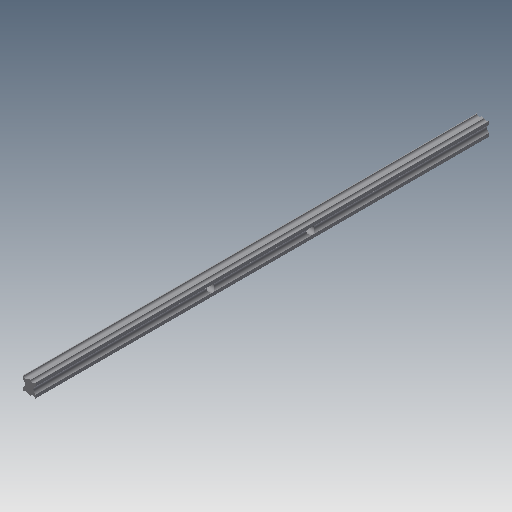
# Autodesk Inventor part: SAR340-40_r
Saved by Autodesk Inventor 2020 (Build 240168000, 168)
## iProperties
Created: 2019-11-23
Part Number: SAR340-40_r
Material: Generic
Catalog Web Link: www.cadenas.de
Description: SAR3_rail-Slide Rails - Aluminum Alloy - Three - Step Slide Rails
Vendor: MISUMI
Document SubType Name: Modeling
Designer: psadmin
Manufacturer: MISUMI
Mass: 40.319 g
Surface Area: 227.079 cm^2
Volume: 40.319 cm^3
Density: 1 g/cm^3
Appearance: PSOLRGB-192-192-192
Category: PARTsolutions
Company: MISUMI
PSOL_IDENT_0: {$CADENAS_DATA\23d-libs\misumi\metric\07_slide_rails\sar3_series\sar3_rail.prj},167 {VTYP=3D},{NB=SA
PSOL_IDENT_1: R340-40_r},{LINA=SAR340-40},{NN=SAR3_rail},{DATE=17.04.2019 06:32:22},{GEOMDATE=16.04.2019 09:30:43}
PSOL_IDENT_2: ,{VERSION=},{LINEID=10},{WBVAR=NO},{WBNUMERIC=NO}  {NB=SAR340-40_r},{LINA=SAR340-40},{KT=DUMMY},{PN=
PSOL_IDENT_3: SAR340-40},{TYPE=SAR340},{MAT1=Aluminum Alloy},{ST1=Clear Anodizing},{MAT2=Aluminum Alloy},{ST2=Clea
PSOL_IDENT_4: r Anodizing},{MAT3=Steel},{NO=40},{RL=400},{TD=460},{A=185},{B=370},{C=185},{D=370},{RLO=147},{BA=36
PSOL_IDENT_5: },{E=156.000},{F=88.000}
NN: SAR3_rail
NT: Slide Rails - Aluminum Alloy - Three - Step Slide Rails
NB: SAR340-40_r
NBSYN: $PN._r
LINA: SAR340-40
PN: SAR340-40
MAT1: Aluminum Alloy
ST1: Clear Anodizing
MAT2: Aluminum Alloy
ST2: Clear Anodizing
MAT3: Steel
NO: 40
RLO: 147
SUPPLIER: MISUMI
ARTICLENO: SAR340-40_r
BOMINFO: SAR340-40
CREATOR: CADENAS GmbH
Title: SAR340-40
Author: Cadenas PARTsolutions
Comments: Slide Rails - Aluminum Alloy - Three - Step Slide Rails
Autodesk Inventor part; units mm, degrees
sketch "_____1" plane through (0, 0, 0) normal (0, 0, 1) x (1, 0, 0)
  arc A0 (0, 0.2) -> (0.2, 0) centre (0.2, 0.2) ccw
  line L0 (0.2, 0) -> (0.5141, 0)
  arc A1 (0.5141, 0) -> (0.708, 0.151) centre (0.5141, 0.2) ccw
  arc A2 (4.392, 0.151) -> (0.708, 0.151) centre (2.55, -0.315) ccw
  arc A3 (4.392, 0.151) -> (4.5859, 0) centre (4.5859, 0.2) ccw
  line L1 (4.5859, 0) -> (6.8141, 0)
  arc A4 (6.8141, 0) -> (7.008, 0.151) centre (6.8141, 0.2) ccw
  arc A5 (10.692, 0.151) -> (7.008, 0.151) centre (8.85, -0.315) ccw
  arc A6 (10.692, 0.151) -> (10.8859, 0) centre (10.8859, 0.2) ccw
  line L2 (10.8859, 0) -> (11.2, 0)
  arc A7 (11.2, 0) -> (11.4, 0.2) centre (11.2, 0.2) ccw
  line L3 (11.4, 0.2) -> (11.4, 2.838)
  arc A8 (11.4, 2.838) -> (11.2882, 3.0174) centre (11.2, 2.838) ccw
  arc A9 (11.2882, 9.0826) -> (11.2882, 3.0174) centre (12.7793, 6.05) ccw
  arc A10 (11.2882, 9.0826) -> (11.4, 9.262) centre (11.2, 9.262) ccw
  line L4 (11.4, 9.262) -> (11.4, 11.9)
  arc A11 (11.4, 11.9) -> (11.2, 12.1) centre (11.2, 11.9) ccw
  line L5 (11.2, 12.1) -> (10.8859, 12.1)
  arc A12 (10.8859, 12.1) -> (10.692, 11.949) centre (10.8859, 11.9) ccw
  arc A13 (7.008, 11.949) -> (10.692, 11.949) centre (8.85, 12.415) ccw
  arc A14 (7.008, 11.949) -> (6.8141, 12.1) centre (6.8141, 11.9) ccw
  line L6 (6.8141, 12.1) -> (4.5859, 12.1)
  arc A15 (4.5859, 12.1) -> (4.392, 11.949) centre (4.5859, 11.9) ccw
  arc A16 (0.708, 11.949) -> (4.392, 11.949) centre (2.55, 12.415) ccw
  arc A17 (0.708, 11.949) -> (0.5141, 12.1) centre (0.5141, 11.9) ccw
  line L7 (0.5141, 12.1) -> (0.2, 12.1)
  arc A18 (0.2, 12.1) -> (0, 11.9) centre (0.2, 11.9) ccw
  line L8 (0, 11.9) -> (0, 9.262)
  arc A19 (0, 9.262) -> (0.1118, 9.0826) centre (0.2, 9.262) ccw
  arc A20 (0.1118, 3.0174) -> (0.1118, 9.0826) centre (-1.3793, 6.05) ccw
  arc A21 (0.1118, 3.0174) -> (0, 2.838) centre (0.2, 2.838) ccw
  line L9 (0, 2.838) -> (0, 0.2)
  constraints: 44 point on circle, 22 centre point, 20 end point
extrude "Extrusion1" add sketch "_____1" along normal blind 400
sketch "Sketch_3" plane through (0, 0, 156) normal (0, 0, 1) x (1, 0, 0)
  line L0 (11.4, 6.05) -> (0, 6.05)
  line L1 (0, 6.05) -> (0, 9.3)
  line L2 (0, 9.3) -> (11.4, 9.3)
  line L3 (11.4, 9.3) -> (11.4, 6.05)
  line L4 (11.4, 6.05) -> (0, 6.05)
  constraints: 10 end point
revolve "Revolution1" cut sketch "Sketch_3" angle 360 about axis through (11.4, 6.05, 156) along (1, 0, 0)
pattern_linear "Rectangular Pattern1" count 2 spacing 88 along (0, 0, 1) of "Revolution1"
ref_plane "to_ball1_1_XY" through (2.55, -0.4, 268.4) normal (0, 1, 0) x (1, 0, 0)
ref_plane "to_ball1_1_YZ" through (2.55, -0.4, 268.4) normal (1, 0, 0) x (0, 0, -1)
ref_plane "to_ball1_1_ZX" through (2.55, -0.4, 268.4) normal (0, 0, -1) x (0, 1, 0)
ref_plane "to_ball1_10_XY" through (2.55, -0.4, 234.2) normal (0, 1, 0) x (1, 0, 0)
ref_plane "to_ball1_10_YZ" through (2.55, -0.4, 234.2) normal (1, 0, 0) x (0, 0, -1)
ref_plane "to_ball1_10_ZX" through (2.55, -0.4, 234.2) normal (0, 0, -1) x (0, 1, 0)
ref_plane "to_ball1_11_XY" through (2.55, -0.4, 230.4) normal (0, 1, 0) x (1, 0, 0)
ref_plane "to_ball1_11_YZ" through (2.55, -0.4, 230.4) normal (1, 0, 0) x (0, 0, -1)
ref_plane "to_ball1_11_ZX" through (2.55, -0.4, 230.4) normal (0, 0, -1) x (0, 1, 0)
ref_plane "to_ball1_12_XY" through (2.55, -0.4, 226.6) normal (0, 1, 0) x (1, 0, 0)
ref_plane "to_ball1_12_YZ" through (2.55, -0.4, 226.6) normal (1, 0, 0) x (0, 0, -1)
ref_plane "to_ball1_12_ZX" through (2.55, -0.4, 226.6) normal (0, 0, -1) x (0, 1, 0)
ref_plane "to_ball1_13_XY" through (2.55, -0.4, 222.8) normal (0, 1, 0) x (1, 0, 0)
ref_plane "to_ball1_13_YZ" through (2.55, -0.4, 222.8) normal (1, 0, 0) x (0, 0, -1)
ref_plane "to_ball1_13_ZX" through (2.55, -0.4, 222.8) normal (0, 0, -1) x (0, 1, 0)
ref_plane "to_ball1_14_XY" through (2.55, -0.4, 219) normal (0, 1, 0) x (1, 0, 0)
ref_plane "to_ball1_14_YZ" through (2.55, -0.4, 219) normal (1, 0, 0) x (0, 0, -1)
ref_plane "to_ball1_14_ZX" through (2.55, -0.4, 219) normal (0, 0, -1) x (0, 1, 0)
ref_plane "to_ball1_15_XY" through (2.55, -0.4, 215.2) normal (0, 1, 0) x (1, 0, 0)
ref_plane "to_ball1_15_YZ" through (2.55, -0.4, 215.2) normal (1, 0, 0) x (0, 0, -1)
ref_plane "to_ball1_15_ZX" through (2.55, -0.4, 215.2) normal (0, 0, -1) x (0, 1, 0)
ref_plane "to_ball1_16_XY" through (2.55, -0.4, 211.4) normal (0, 1, 0) x (1, 0, 0)
ref_plane "to_ball1_16_YZ" through (2.55, -0.4, 211.4) normal (1, 0, 0) x (0, 0, -1)
ref_plane "to_ball1_16_ZX" through (2.55, -0.4, 211.4) normal (0, 0, -1) x (0, 1, 0)
ref_plane "to_ball1_17_XY" through (2.55, -0.4, 207.6) normal (0, 1, 0) x (1, 0, 0)
ref_plane "to_ball1_17_YZ" through (2.55, -0.4, 207.6) normal (1, 0, 0) x (0, 0, -1)
ref_plane "to_ball1_17_ZX" through (2.55, -0.4, 207.6) normal (0, 0, -1) x (0, 1, 0)
ref_plane "to_ball1_18_XY" through (2.55, -0.4, 203.8) normal (0, 1, 0) x (1, 0, 0)
ref_plane "to_ball1_18_YZ" through (2.55, -0.4, 203.8) normal (1, 0, 0) x (0, 0, -1)
ref_plane "to_ball1_18_ZX" through (2.55, -0.4, 203.8) normal (0, 0, -1) x (0, 1, 0)
ref_plane "to_ball1_19_XY" through (2.55, -0.4, 200) normal (0, 1, 0) x (1, 0, 0)
ref_plane "to_ball1_19_YZ" through (2.55, -0.4, 200) normal (1, 0, 0) x (0, 0, -1)
ref_plane "to_ball1_19_ZX" through (2.55, -0.4, 200) normal (0, 0, -1) x (0, 1, 0)
ref_plane "to_ball1_2_XY" through (2.55, -0.4, 264.6) normal (0, 1, 0) x (1, 0, 0)
ref_plane "to_ball1_2_YZ" through (2.55, -0.4, 264.6) normal (1, 0, 0) x (0, 0, -1)
ref_plane "to_ball1_2_ZX" through (2.55, -0.4, 264.6) normal (0, 0, -1) x (0, 1, 0)
ref_plane "to_ball1_20_XY" through (2.55, -0.4, 196.2) normal (0, 1, 0) x (1, 0, 0)
ref_plane "to_ball1_20_YZ" through (2.55, -0.4, 196.2) normal (1, 0, 0) x (0, 0, -1)
ref_plane "to_ball1_20_ZX" through (2.55, -0.4, 196.2) normal (0, 0, -1) x (0, 1, 0)
ref_plane "to_ball1_21_XY" through (2.55, -0.4, 192.4) normal (0, 1, 0) x (1, 0, 0)
ref_plane "to_ball1_21_YZ" through (2.55, -0.4, 192.4) normal (1, 0, 0) x (0, 0, -1)
ref_plane "to_ball1_21_ZX" through (2.55, -0.4, 192.4) normal (0, 0, -1) x (0, 1, 0)
ref_plane "to_ball1_22_XY" through (2.55, -0.4, 188.6) normal (0, 1, 0) x (1, 0, 0)
ref_plane "to_ball1_22_YZ" through (2.55, -0.4, 188.6) normal (1, 0, 0) x (0, 0, -1)
ref_plane "to_ball1_22_ZX" through (2.55, -0.4, 188.6) normal (0, 0, -1) x (0, 1, 0)
ref_plane "to_ball1_23_XY" through (2.55, -0.4, 184.8) normal (0, 1, 0) x (1, 0, 0)
ref_plane "to_ball1_23_YZ" through (2.55, -0.4, 184.8) normal (1, 0, 0) x (0, 0, -1)
ref_plane "to_ball1_23_ZX" through (2.55, -0.4, 184.8) normal (0, 0, -1) x (0, 1, 0)
ref_plane "to_ball1_24_XY" through (2.55, -0.4, 181) normal (0, 1, 0) x (1, 0, 0)
ref_plane "to_ball1_24_YZ" through (2.55, -0.4, 181) normal (1, 0, 0) x (0, 0, -1)
ref_plane "to_ball1_24_ZX" through (2.55, -0.4, 181) normal (0, 0, -1) x (0, 1, 0)
ref_plane "to_ball1_25_XY" through (2.55, -0.4, 177.2) normal (0, 1, 0) x (1, 0, 0)
ref_plane "to_ball1_25_YZ" through (2.55, -0.4, 177.2) normal (1, 0, 0) x (0, 0, -1)
ref_plane "to_ball1_25_ZX" through (2.55, -0.4, 177.2) normal (0, 0, -1) x (0, 1, 0)
ref_plane "to_ball1_26_XY" through (2.55, -0.4, 173.4) normal (0, 1, 0) x (1, 0, 0)
ref_plane "to_ball1_26_YZ" through (2.55, -0.4, 173.4) normal (1, 0, 0) x (0, 0, -1)
ref_plane "to_ball1_26_ZX" through (2.55, -0.4, 173.4) normal (0, 0, -1) x (0, 1, 0)
ref_plane "to_ball1_27_XY" through (2.55, -0.4, 169.6) normal (0, 1, 0) x (1, 0, 0)
ref_plane "to_ball1_27_YZ" through (2.55, -0.4, 169.6) normal (1, 0, 0) x (0, 0, -1)
ref_plane "to_ball1_27_ZX" through (2.55, -0.4, 169.6) normal (0, 0, -1) x (0, 1, 0)
ref_plane "to_ball1_28_XY" through (2.55, -0.4, 165.8) normal (0, 1, 0) x (1, 0, 0)
ref_plane "to_ball1_28_YZ" through (2.55, -0.4, 165.8) normal (1, 0, 0) x (0, 0, -1)
ref_plane "to_ball1_28_ZX" through (2.55, -0.4, 165.8) normal (0, 0, -1) x (0, 1, 0)
ref_plane "to_ball1_29_XY" through (2.55, -0.4, 162) normal (0, 1, 0) x (1, 0, 0)
ref_plane "to_ball1_29_YZ" through (2.55, -0.4, 162) normal (1, 0, 0) x (0, 0, -1)
ref_plane "to_ball1_29_ZX" through (2.55, -0.4, 162) normal (0, 0, -1) x (0, 1, 0)
ref_plane "to_ball1_3_XY" through (2.55, -0.4, 260.8) normal (0, 1, 0) x (1, 0, 0)
ref_plane "to_ball1_3_YZ" through (2.55, -0.4, 260.8) normal (1, 0, 0) x (0, 0, -1)
ref_plane "to_ball1_3_ZX" through (2.55, -0.4, 260.8) normal (0, 0, -1) x (0, 1, 0)
ref_plane "to_ball1_30_XY" through (2.55, -0.4, 158.2) normal (0, 1, 0) x (1, 0, 0)
ref_plane "to_ball1_30_YZ" through (2.55, -0.4, 158.2) normal (1, 0, 0) x (0, 0, -1)
ref_plane "to_ball1_30_ZX" through (2.55, -0.4, 158.2) normal (0, 0, -1) x (0, 1, 0)
ref_plane "to_ball1_31_XY" through (2.55, -0.4, 154.4) normal (0, 1, 0) x (1, 0, 0)
ref_plane "to_ball1_31_YZ" through (2.55, -0.4, 154.4) normal (1, 0, 0) x (0, 0, -1)
ref_plane "to_ball1_31_ZX" through (2.55, -0.4, 154.4) normal (0, 0, -1) x (0, 1, 0)
ref_plane "to_ball1_32_XY" through (2.55, -0.4, 150.6) normal (0, 1, 0) x (1, 0, 0)
ref_plane "to_ball1_32_YZ" through (2.55, -0.4, 150.6) normal (1, 0, 0) x (0, 0, -1)
ref_plane "to_ball1_32_ZX" through (2.55, -0.4, 150.6) normal (0, 0, -1) x (0, 1, 0)
ref_plane "to_ball1_33_XY" through (2.55, -0.4, 146.8) normal (0, 1, 0) x (1, 0, 0)
ref_plane "to_ball1_33_YZ" through (2.55, -0.4, 146.8) normal (1, 0, 0) x (0, 0, -1)
ref_plane "to_ball1_33_ZX" through (2.55, -0.4, 146.8) normal (0, 0, -1) x (0, 1, 0)
ref_plane "to_ball1_34_XY" through (2.55, -0.4, 143) normal (0, 1, 0) x (1, 0, 0)
ref_plane "to_ball1_34_YZ" through (2.55, -0.4, 143) normal (1, 0, 0) x (0, 0, -1)
ref_plane "to_ball1_34_ZX" through (2.55, -0.4, 143) normal (0, 0, -1) x (0, 1, 0)
ref_plane "to_ball1_35_XY" through (2.55, -0.4, 139.2) normal (0, 1, 0) x (1, 0, 0)
ref_plane "to_ball1_35_YZ" through (2.55, -0.4, 139.2) normal (1, 0, 0) x (0, 0, -1)
ref_plane "to_ball1_35_ZX" through (2.55, -0.4, 139.2) normal (0, 0, -1) x (0, 1, 0)
ref_plane "to_ball1_36_XY" through (2.55, -0.4, 135.4) normal (0, 1, 0) x (1, 0, 0)
ref_plane "to_ball1_36_YZ" through (2.55, -0.4, 135.4) normal (1, 0, 0) x (0, 0, -1)
ref_plane "to_ball1_36_ZX" through (2.55, -0.4, 135.4) normal (0, 0, -1) x (0, 1, 0)
ref_plane "to_ball1_37_XY" through (2.55, -0.4, 131.6) normal (0, 1, 0) x (1, 0, 0)
ref_plane "to_ball1_37_YZ" through (2.55, -0.4, 131.6) normal (1, 0, 0) x (0, 0, -1)
ref_plane "to_ball1_37_ZX" through (2.55, -0.4, 131.6) normal (0, 0, -1) x (0, 1, 0)
ref_plane "to_ball1_4_XY" through (2.55, -0.4, 257) normal (0, 1, 0) x (1, 0, 0)
ref_plane "to_ball1_4_YZ" through (2.55, -0.4, 257) normal (1, 0, 0) x (0, 0, -1)
ref_plane "to_ball1_4_ZX" through (2.55, -0.4, 257) normal (0, 0, -1) x (0, 1, 0)
ref_plane "to_ball1_5_XY" through (2.55, -0.4, 253.2) normal (0, 1, 0) x (1, 0, 0)
ref_plane "to_ball1_5_YZ" through (2.55, -0.4, 253.2) normal (1, 0, 0) x (0, 0, -1)
ref_plane "to_ball1_5_ZX" through (2.55, -0.4, 253.2) normal (0, 0, -1) x (0, 1, 0)
ref_plane "to_ball1_6_XY" through (2.55, -0.4, 249.4) normal (0, 1, 0) x (1, 0, 0)
ref_plane "to_ball1_6_YZ" through (2.55, -0.4, 249.4) normal (1, 0, 0) x (0, 0, -1)
ref_plane "to_ball1_6_ZX" through (2.55, -0.4, 249.4) normal (0, 0, -1) x (0, 1, 0)
ref_plane "to_ball1_7_XY" through (2.55, -0.4, 245.6) normal (0, 1, 0) x (1, 0, 0)
ref_plane "to_ball1_7_YZ" through (2.55, -0.4, 245.6) normal (1, 0, 0) x (0, 0, -1)
ref_plane "to_ball1_7_ZX" through (2.55, -0.4, 245.6) normal (0, 0, -1) x (0, 1, 0)
ref_plane "to_ball1_8_XY" through (2.55, -0.4, 241.8) normal (0, 1, 0) x (1, 0, 0)
ref_plane "to_ball1_8_YZ" through (2.55, -0.4, 241.8) normal (1, 0, 0) x (0, 0, -1)
ref_plane "to_ball1_8_ZX" through (2.55, -0.4, 241.8) normal (0, 0, -1) x (0, 1, 0)
ref_plane "to_ball1_9_XY" through (2.55, -0.4, 238) normal (0, 1, 0) x (1, 0, 0)
ref_plane "to_ball1_9_YZ" through (2.55, -0.4, 238) normal (1, 0, 0) x (0, 0, -1)
ref_plane "to_ball1_9_ZX" through (2.55, -0.4, 238) normal (0, 0, -1) x (0, 1, 0)
ref_plane "to_ball2_1_XY" through (8.85, -0.4, 268.4) normal (0, 1, 0) x (1, 0, 0)
ref_plane "to_ball2_1_YZ" through (8.85, -0.4, 268.4) normal (1, 0, 0) x (0, 0, -1)
ref_plane "to_ball2_1_ZX" through (8.85, -0.4, 268.4) normal (0, 0, -1) x (0, 1, 0)
ref_plane "to_ball2_10_XY" through (8.85, -0.4, 234.2) normal (0, 1, 0) x (1, 0, 0)
ref_plane "to_ball2_10_YZ" through (8.85, -0.4, 234.2) normal (1, 0, 0) x (0, 0, -1)
ref_plane "to_ball2_10_ZX" through (8.85, -0.4, 234.2) normal (0, 0, -1) x (0, 1, 0)
ref_plane "to_ball2_11_XY" through (8.85, -0.4, 230.4) normal (0, 1, 0) x (1, 0, 0)
ref_plane "to_ball2_11_YZ" through (8.85, -0.4, 230.4) normal (1, 0, 0) x (0, 0, -1)
ref_plane "to_ball2_11_ZX" through (8.85, -0.4, 230.4) normal (0, 0, -1) x (0, 1, 0)
ref_plane "to_ball2_12_XY" through (8.85, -0.4, 226.6) normal (0, 1, 0) x (1, 0, 0)
ref_plane "to_ball2_12_YZ" through (8.85, -0.4, 226.6) normal (1, 0, 0) x (0, 0, -1)
ref_plane "to_ball2_12_ZX" through (8.85, -0.4, 226.6) normal (0, 0, -1) x (0, 1, 0)
ref_plane "to_ball2_13_XY" through (8.85, -0.4, 222.8) normal (0, 1, 0) x (1, 0, 0)
ref_plane "to_ball2_13_YZ" through (8.85, -0.4, 222.8) normal (1, 0, 0) x (0, 0, -1)
ref_plane "to_ball2_13_ZX" through (8.85, -0.4, 222.8) normal (0, 0, -1) x (0, 1, 0)
ref_plane "to_ball2_14_XY" through (8.85, -0.4, 219) normal (0, 1, 0) x (1, 0, 0)
ref_plane "to_ball2_14_YZ" through (8.85, -0.4, 219) normal (1, 0, 0) x (0, 0, -1)
ref_plane "to_ball2_14_ZX" through (8.85, -0.4, 219) normal (0, 0, -1) x (0, 1, 0)
ref_plane "to_ball2_15_XY" through (8.85, -0.4, 215.2) normal (0, 1, 0) x (1, 0, 0)
ref_plane "to_ball2_15_YZ" through (8.85, -0.4, 215.2) normal (1, 0, 0) x (0, 0, -1)
ref_plane "to_ball2_15_ZX" through (8.85, -0.4, 215.2) normal (0, 0, -1) x (0, 1, 0)
ref_plane "to_ball2_16_XY" through (8.85, -0.4, 211.4) normal (0, 1, 0) x (1, 0, 0)
ref_plane "to_ball2_16_YZ" through (8.85, -0.4, 211.4) normal (1, 0, 0) x (0, 0, -1)
ref_plane "to_ball2_16_ZX" through (8.85, -0.4, 211.4) normal (0, 0, -1) x (0, 1, 0)
ref_plane "to_ball2_17_XY" through (8.85, -0.4, 207.6) normal (0, 1, 0) x (1, 0, 0)
ref_plane "to_ball2_17_YZ" through (8.85, -0.4, 207.6) normal (1, 0, 0) x (0, 0, -1)
ref_plane "to_ball2_17_ZX" through (8.85, -0.4, 207.6) normal (0, 0, -1) x (0, 1, 0)
ref_plane "to_ball2_18_XY" through (8.85, -0.4, 203.8) normal (0, 1, 0) x (1, 0, 0)
ref_plane "to_ball2_18_YZ" through (8.85, -0.4, 203.8) normal (1, 0, 0) x (0, 0, -1)
ref_plane "to_ball2_18_ZX" through (8.85, -0.4, 203.8) normal (0, 0, -1) x (0, 1, 0)
ref_plane "to_ball2_19_XY" through (8.85, -0.4, 200) normal (0, 1, 0) x (1, 0, 0)
ref_plane "to_ball2_19_YZ" through (8.85, -0.4, 200) normal (1, 0, 0) x (0, 0, -1)
ref_plane "to_ball2_19_ZX" through (8.85, -0.4, 200) normal (0, 0, -1) x (0, 1, 0)
ref_plane "to_ball2_2_XY" through (8.85, -0.4, 264.6) normal (0, 1, 0) x (1, 0, 0)
ref_plane "to_ball2_2_YZ" through (8.85, -0.4, 264.6) normal (1, 0, 0) x (0, 0, -1)
ref_plane "to_ball2_2_ZX" through (8.85, -0.4, 264.6) normal (0, 0, -1) x (0, 1, 0)
ref_plane "to_ball2_20_XY" through (8.85, -0.4, 196.2) normal (0, 1, 0) x (1, 0, 0)
ref_plane "to_ball2_20_YZ" through (8.85, -0.4, 196.2) normal (1, 0, 0) x (0, 0, -1)
ref_plane "to_ball2_20_ZX" through (8.85, -0.4, 196.2) normal (0, 0, -1) x (0, 1, 0)
ref_plane "to_ball2_21_XY" through (8.85, -0.4, 192.4) normal (0, 1, 0) x (1, 0, 0)
ref_plane "to_ball2_21_YZ" through (8.85, -0.4, 192.4) normal (1, 0, 0) x (0, 0, -1)
ref_plane "to_ball2_21_ZX" through (8.85, -0.4, 192.4) normal (0, 0, -1) x (0, 1, 0)
ref_plane "to_ball2_22_XY" through (8.85, -0.4, 188.6) normal (0, 1, 0) x (1, 0, 0)
ref_plane "to_ball2_22_YZ" through (8.85, -0.4, 188.6) normal (1, 0, 0) x (0, 0, -1)
ref_plane "to_ball2_22_ZX" through (8.85, -0.4, 188.6) normal (0, 0, -1) x (0, 1, 0)
ref_plane "to_ball2_23_XY" through (8.85, -0.4, 184.8) normal (0, 1, 0) x (1, 0, 0)
ref_plane "to_ball2_23_YZ" through (8.85, -0.4, 184.8) normal (1, 0, 0) x (0, 0, -1)
ref_plane "to_ball2_23_ZX" through (8.85, -0.4, 184.8) normal (0, 0, -1) x (0, 1, 0)
ref_plane "to_ball2_24_XY" through (8.85, -0.4, 181) normal (0, 1, 0) x (1, 0, 0)
ref_plane "to_ball2_24_YZ" through (8.85, -0.4, 181) normal (1, 0, 0) x (0, 0, -1)
ref_plane "to_ball2_24_ZX" through (8.85, -0.4, 181) normal (0, 0, -1) x (0, 1, 0)
ref_plane "to_ball2_25_XY" through (8.85, -0.4, 177.2) normal (0, 1, 0) x (1, 0, 0)
ref_plane "to_ball2_25_YZ" through (8.85, -0.4, 177.2) normal (1, 0, 0) x (0, 0, -1)
ref_plane "to_ball2_25_ZX" through (8.85, -0.4, 177.2) normal (0, 0, -1) x (0, 1, 0)
ref_plane "to_ball2_26_XY" through (8.85, -0.4, 173.4) normal (0, 1, 0) x (1, 0, 0)
ref_plane "to_ball2_26_YZ" through (8.85, -0.4, 173.4) normal (1, 0, 0) x (0, 0, -1)
ref_plane "to_ball2_26_ZX" through (8.85, -0.4, 173.4) normal (0, 0, -1) x (0, 1, 0)
ref_plane "to_ball2_27_XY" through (8.85, -0.4, 169.6) normal (0, 1, 0) x (1, 0, 0)
ref_plane "to_ball2_27_YZ" through (8.85, -0.4, 169.6) normal (1, 0, 0) x (0, 0, -1)
ref_plane "to_ball2_27_ZX" through (8.85, -0.4, 169.6) normal (0, 0, -1) x (0, 1, 0)
ref_plane "to_ball2_28_XY" through (8.85, -0.4, 165.8) normal (0, 1, 0) x (1, 0, 0)
ref_plane "to_ball2_28_YZ" through (8.85, -0.4, 165.8) normal (1, 0, 0) x (0, 0, -1)
ref_plane "to_ball2_28_ZX" through (8.85, -0.4, 165.8) normal (0, 0, -1) x (0, 1, 0)
ref_plane "to_ball2_29_XY" through (8.85, -0.4, 162) normal (0, 1, 0) x (1, 0, 0)
ref_plane "to_ball2_29_YZ" through (8.85, -0.4, 162) normal (1, 0, 0) x (0, 0, -1)
ref_plane "to_ball2_29_ZX" through (8.85, -0.4, 162) normal (0, 0, -1) x (0, 1, 0)
ref_plane "to_ball2_3_XY" through (8.85, -0.4, 260.8) normal (0, 1, 0) x (1, 0, 0)
ref_plane "to_ball2_3_YZ" through (8.85, -0.4, 260.8) normal (1, 0, 0) x (0, 0, -1)
ref_plane "to_ball2_3_ZX" through (8.85, -0.4, 260.8) normal (0, 0, -1) x (0, 1, 0)
ref_plane "to_ball2_30_XY" through (8.85, -0.4, 158.2) normal (0, 1, 0) x (1, 0, 0)
ref_plane "to_ball2_30_YZ" through (8.85, -0.4, 158.2) normal (1, 0, 0) x (0, 0, -1)
ref_plane "to_ball2_30_ZX" through (8.85, -0.4, 158.2) normal (0, 0, -1) x (0, 1, 0)
ref_plane "to_ball2_31_XY" through (8.85, -0.4, 154.4) normal (0, 1, 0) x (1, 0, 0)
ref_plane "to_ball2_31_YZ" through (8.85, -0.4, 154.4) normal (1, 0, 0) x (0, 0, -1)
ref_plane "to_ball2_31_ZX" through (8.85, -0.4, 154.4) normal (0, 0, -1) x (0, 1, 0)
ref_plane "to_ball2_32_XY" through (8.85, -0.4, 150.6) normal (0, 1, 0) x (1, 0, 0)
ref_plane "to_ball2_32_YZ" through (8.85, -0.4, 150.6) normal (1, 0, 0) x (0, 0, -1)
ref_plane "to_ball2_32_ZX" through (8.85, -0.4, 150.6) normal (0, 0, -1) x (0, 1, 0)
ref_plane "to_ball2_33_XY" through (8.85, -0.4, 146.8) normal (0, 1, 0) x (1, 0, 0)
ref_plane "to_ball2_33_YZ" through (8.85, -0.4, 146.8) normal (1, 0, 0) x (0, 0, -1)
ref_plane "to_ball2_33_ZX" through (8.85, -0.4, 146.8) normal (0, 0, -1) x (0, 1, 0)
ref_plane "to_ball2_34_XY" through (8.85, -0.4, 143) normal (0, 1, 0) x (1, 0, 0)
ref_plane "to_ball2_34_YZ" through (8.85, -0.4, 143) normal (1, 0, 0) x (0, 0, -1)
ref_plane "to_ball2_34_ZX" through (8.85, -0.4, 143) normal (0, 0, -1) x (0, 1, 0)
ref_plane "to_ball2_35_XY" through (8.85, -0.4, 139.2) normal (0, 1, 0) x (1, 0, 0)
ref_plane "to_ball2_35_YZ" through (8.85, -0.4, 139.2) normal (1, 0, 0) x (0, 0, -1)
ref_plane "to_ball2_35_ZX" through (8.85, -0.4, 139.2) normal (0, 0, -1) x (0, 1, 0)
ref_plane "to_ball2_36_XY" through (8.85, -0.4, 135.4) normal (0, 1, 0) x (1, 0, 0)
ref_plane "to_ball2_36_YZ" through (8.85, -0.4, 135.4) normal (1, 0, 0) x (0, 0, -1)
ref_plane "to_ball2_36_ZX" through (8.85, -0.4, 135.4) normal (0, 0, -1) x (0, 1, 0)
ref_plane "to_ball2_37_XY" through (8.85, -0.4, 131.6) normal (0, 1, 0) x (1, 0, 0)
ref_plane "to_ball2_37_YZ" through (8.85, -0.4, 131.6) normal (1, 0, 0) x (0, 0, -1)
ref_plane "to_ball2_37_ZX" through (8.85, -0.4, 131.6) normal (0, 0, -1) x (0, 1, 0)
ref_plane "to_ball2_4_XY" through (8.85, -0.4, 257) normal (0, 1, 0) x (1, 0, 0)
ref_plane "to_ball2_4_YZ" through (8.85, -0.4, 257) normal (1, 0, 0) x (0, 0, -1)
ref_plane "to_ball2_4_ZX" through (8.85, -0.4, 257) normal (0, 0, -1) x (0, 1, 0)
ref_plane "to_ball2_5_XY" through (8.85, -0.4, 253.2) normal (0, 1, 0) x (1, 0, 0)
ref_plane "to_ball2_5_YZ" through (8.85, -0.4, 253.2) normal (1, 0, 0) x (0, 0, -1)
ref_plane "to_ball2_5_ZX" through (8.85, -0.4, 253.2) normal (0, 0, -1) x (0, 1, 0)
ref_plane "to_ball2_6_XY" through (8.85, -0.4, 249.4) normal (0, 1, 0) x (1, 0, 0)
ref_plane "to_ball2_6_YZ" through (8.85, -0.4, 249.4) normal (1, 0, 0) x (0, 0, -1)
ref_plane "to_ball2_6_ZX" through (8.85, -0.4, 249.4) normal (0, 0, -1) x (0, 1, 0)
ref_plane "to_ball2_7_XY" through (8.85, -0.4, 245.6) normal (0, 1, 0) x (1, 0, 0)
ref_plane "to_ball2_7_YZ" through (8.85, -0.4, 245.6) normal (1, 0, 0) x (0, 0, -1)
ref_plane "to_ball2_7_ZX" through (8.85, -0.4, 245.6) normal (0, 0, -1) x (0, 1, 0)
ref_plane "to_ball2_8_XY" through (8.85, -0.4, 241.8) normal (0, 1, 0) x (1, 0, 0)
ref_plane "to_ball2_8_YZ" through (8.85, -0.4, 241.8) normal (1, 0, 0) x (0, 0, -1)
ref_plane "to_ball2_8_ZX" through (8.85, -0.4, 241.8) normal (0, 0, -1) x (0, 1, 0)
ref_plane "to_ball2_9_XY" through (8.85, -0.4, 238) normal (0, 1, 0) x (1, 0, 0)
ref_plane "to_ball2_9_YZ" through (8.85, -0.4, 238) normal (1, 0, 0) x (0, 0, -1)
ref_plane "to_ball2_9_ZX" through (8.85, -0.4, 238) normal (0, 0, -1) x (0, 1, 0)
ref_plane "to_ball3_1_XY" through (2.55, 12.5, 268.4) normal (0, 1, 0) x (1, 0, 0)
ref_plane "to_ball3_1_YZ" through (2.55, 12.5, 268.4) normal (1, 0, 0) x (0, 0, -1)
ref_plane "to_ball3_1_ZX" through (2.55, 12.5, 268.4) normal (0, 0, -1) x (0, 1, 0)
ref_plane "to_ball3_10_XY" through (2.55, 12.5, 234.2) normal (0, 1, 0) x (1, 0, 0)
ref_plane "to_ball3_10_YZ" through (2.55, 12.5, 234.2) normal (1, 0, 0) x (0, 0, -1)
ref_plane "to_ball3_10_ZX" through (2.55, 12.5, 234.2) normal (0, 0, -1) x (0, 1, 0)
ref_plane "to_ball3_11_XY" through (2.55, 12.5, 230.4) normal (0, 1, 0) x (1, 0, 0)
ref_plane "to_ball3_11_YZ" through (2.55, 12.5, 230.4) normal (1, 0, 0) x (0, 0, -1)
ref_plane "to_ball3_11_ZX" through (2.55, 12.5, 230.4) normal (0, 0, -1) x (0, 1, 0)
ref_plane "to_ball3_12_XY" through (2.55, 12.5, 226.6) normal (0, 1, 0) x (1, 0, 0)
ref_plane "to_ball3_12_YZ" through (2.55, 12.5, 226.6) normal (1, 0, 0) x (0, 0, -1)
ref_plane "to_ball3_12_ZX" through (2.55, 12.5, 226.6) normal (0, 0, -1) x (0, 1, 0)
ref_plane "to_ball3_13_XY" through (2.55, 12.5, 222.8) normal (0, 1, 0) x (1, 0, 0)
ref_plane "to_ball3_13_YZ" through (2.55, 12.5, 222.8) normal (1, 0, 0) x (0, 0, -1)
ref_plane "to_ball3_13_ZX" through (2.55, 12.5, 222.8) normal (0, 0, -1) x (0, 1, 0)
ref_plane "to_ball3_14_XY" through (2.55, 12.5, 219) normal (0, 1, 0) x (1, 0, 0)
ref_plane "to_ball3_14_YZ" through (2.55, 12.5, 219) normal (1, 0, 0) x (0, 0, -1)
ref_plane "to_ball3_14_ZX" through (2.55, 12.5, 219) normal (0, 0, -1) x (0, 1, 0)
ref_plane "to_ball3_15_XY" through (2.55, 12.5, 215.2) normal (0, 1, 0) x (1, 0, 0)
ref_plane "to_ball3_15_YZ" through (2.55, 12.5, 215.2) normal (1, 0, 0) x (0, 0, -1)
ref_plane "to_ball3_15_ZX" through (2.55, 12.5, 215.2) normal (0, 0, -1) x (0, 1, 0)
ref_plane "to_ball3_16_XY" through (2.55, 12.5, 211.4) normal (0, 1, 0) x (1, 0, 0)
ref_plane "to_ball3_16_YZ" through (2.55, 12.5, 211.4) normal (1, 0, 0) x (0, 0, -1)
ref_plane "to_ball3_16_ZX" through (2.55, 12.5, 211.4) normal (0, 0, -1) x (0, 1, 0)
ref_plane "to_ball3_17_XY" through (2.55, 12.5, 207.6) normal (0, 1, 0) x (1, 0, 0)
ref_plane "to_ball3_17_YZ" through (2.55, 12.5, 207.6) normal (1, 0, 0) x (0, 0, -1)
ref_plane "to_ball3_17_ZX" through (2.55, 12.5, 207.6) normal (0, 0, -1) x (0, 1, 0)
ref_plane "to_ball3_18_XY" through (2.55, 12.5, 203.8) normal (0, 1, 0) x (1, 0, 0)
ref_plane "to_ball3_18_YZ" through (2.55, 12.5, 203.8) normal (1, 0, 0) x (0, 0, -1)
ref_plane "to_ball3_18_ZX" through (2.55, 12.5, 203.8) normal (0, 0, -1) x (0, 1, 0)
ref_plane "to_ball3_19_XY" through (2.55, 12.5, 200) normal (0, 1, 0) x (1, 0, 0)
ref_plane "to_ball3_19_YZ" through (2.55, 12.5, 200) normal (1, 0, 0) x (0, 0, -1)
ref_plane "to_ball3_19_ZX" through (2.55, 12.5, 200) normal (0, 0, -1) x (0, 1, 0)
ref_plane "to_ball3_2_XY" through (2.55, 12.5, 264.6) normal (0, 1, 0) x (1, 0, 0)
ref_plane "to_ball3_2_YZ" through (2.55, 12.5, 264.6) normal (1, 0, 0) x (0, 0, -1)
ref_plane "to_ball3_2_ZX" through (2.55, 12.5, 264.6) normal (0, 0, -1) x (0, 1, 0)
ref_plane "to_ball3_20_XY" through (2.55, 12.5, 196.2) normal (0, 1, 0) x (1, 0, 0)
ref_plane "to_ball3_20_YZ" through (2.55, 12.5, 196.2) normal (1, 0, 0) x (0, 0, -1)
ref_plane "to_ball3_20_ZX" through (2.55, 12.5, 196.2) normal (0, 0, -1) x (0, 1, 0)
ref_plane "to_ball3_21_XY" through (2.55, 12.5, 192.4) normal (0, 1, 0) x (1, 0, 0)
ref_plane "to_ball3_21_YZ" through (2.55, 12.5, 192.4) normal (1, 0, 0) x (0, 0, -1)
ref_plane "to_ball3_21_ZX" through (2.55, 12.5, 192.4) normal (0, 0, -1) x (0, 1, 0)
ref_plane "to_ball3_22_XY" through (2.55, 12.5, 188.6) normal (0, 1, 0) x (1, 0, 0)
ref_plane "to_ball3_22_YZ" through (2.55, 12.5, 188.6) normal (1, 0, 0) x (0, 0, -1)
ref_plane "to_ball3_22_ZX" through (2.55, 12.5, 188.6) normal (0, 0, -1) x (0, 1, 0)
ref_plane "to_ball3_23_XY" through (2.55, 12.5, 184.8) normal (0, 1, 0) x (1, 0, 0)
ref_plane "to_ball3_23_YZ" through (2.55, 12.5, 184.8) normal (1, 0, 0) x (0, 0, -1)
ref_plane "to_ball3_23_ZX" through (2.55, 12.5, 184.8) normal (0, 0, -1) x (0, 1, 0)
ref_plane "to_ball3_24_XY" through (2.55, 12.5, 181) normal (0, 1, 0) x (1, 0, 0)
ref_plane "to_ball3_24_YZ" through (2.55, 12.5, 181) normal (1, 0, 0) x (0, 0, -1)
ref_plane "to_ball3_24_ZX" through (2.55, 12.5, 181) normal (0, 0, -1) x (0, 1, 0)
ref_plane "to_ball3_25_XY" through (2.55, 12.5, 177.2) normal (0, 1, 0) x (1, 0, 0)
ref_plane "to_ball3_25_YZ" through (2.55, 12.5, 177.2) normal (1, 0, 0) x (0, 0, -1)
ref_plane "to_ball3_25_ZX" through (2.55, 12.5, 177.2) normal (0, 0, -1) x (0, 1, 0)
ref_plane "to_ball3_26_XY" through (2.55, 12.5, 173.4) normal (0, 1, 0) x (1, 0, 0)
ref_plane "to_ball3_26_YZ" through (2.55, 12.5, 173.4) normal (1, 0, 0) x (0, 0, -1)
ref_plane "to_ball3_26_ZX" through (2.55, 12.5, 173.4) normal (0, 0, -1) x (0, 1, 0)
ref_plane "to_ball3_27_XY" through (2.55, 12.5, 169.6) normal (0, 1, 0) x (1, 0, 0)
ref_plane "to_ball3_27_YZ" through (2.55, 12.5, 169.6) normal (1, 0, 0) x (0, 0, -1)
ref_plane "to_ball3_27_ZX" through (2.55, 12.5, 169.6) normal (0, 0, -1) x (0, 1, 0)
ref_plane "to_ball3_28_XY" through (2.55, 12.5, 165.8) normal (0, 1, 0) x (1, 0, 0)
ref_plane "to_ball3_28_YZ" through (2.55, 12.5, 165.8) normal (1, 0, 0) x (0, 0, -1)
ref_plane "to_ball3_28_ZX" through (2.55, 12.5, 165.8) normal (0, 0, -1) x (0, 1, 0)
ref_plane "to_ball3_29_XY" through (2.55, 12.5, 162) normal (0, 1, 0) x (1, 0, 0)
ref_plane "to_ball3_29_YZ" through (2.55, 12.5, 162) normal (1, 0, 0) x (0, 0, -1)
ref_plane "to_ball3_29_ZX" through (2.55, 12.5, 162) normal (0, 0, -1) x (0, 1, 0)
ref_plane "to_ball3_3_XY" through (2.55, 12.5, 260.8) normal (0, 1, 0) x (1, 0, 0)
ref_plane "to_ball3_3_YZ" through (2.55, 12.5, 260.8) normal (1, 0, 0) x (0, 0, -1)
ref_plane "to_ball3_3_ZX" through (2.55, 12.5, 260.8) normal (0, 0, -1) x (0, 1, 0)
ref_plane "to_ball3_30_XY" through (2.55, 12.5, 158.2) normal (0, 1, 0) x (1, 0, 0)
ref_plane "to_ball3_30_YZ" through (2.55, 12.5, 158.2) normal (1, 0, 0) x (0, 0, -1)
ref_plane "to_ball3_30_ZX" through (2.55, 12.5, 158.2) normal (0, 0, -1) x (0, 1, 0)
ref_plane "to_ball3_31_XY" through (2.55, 12.5, 154.4) normal (0, 1, 0) x (1, 0, 0)
ref_plane "to_ball3_31_YZ" through (2.55, 12.5, 154.4) normal (1, 0, 0) x (0, 0, -1)
ref_plane "to_ball3_31_ZX" through (2.55, 12.5, 154.4) normal (0, 0, -1) x (0, 1, 0)
ref_plane "to_ball3_32_XY" through (2.55, 12.5, 150.6) normal (0, 1, 0) x (1, 0, 0)
ref_plane "to_ball3_32_YZ" through (2.55, 12.5, 150.6) normal (1, 0, 0) x (0, 0, -1)
ref_plane "to_ball3_32_ZX" through (2.55, 12.5, 150.6) normal (0, 0, -1) x (0, 1, 0)
ref_plane "to_ball3_33_XY" through (2.55, 12.5, 146.8) normal (0, 1, 0) x (1, 0, 0)
ref_plane "to_ball3_33_YZ" through (2.55, 12.5, 146.8) normal (1, 0, 0) x (0, 0, -1)
ref_plane "to_ball3_33_ZX" through (2.55, 12.5, 146.8) normal (0, 0, -1) x (0, 1, 0)
ref_plane "to_ball3_34_XY" through (2.55, 12.5, 143) normal (0, 1, 0) x (1, 0, 0)
ref_plane "to_ball3_34_YZ" through (2.55, 12.5, 143) normal (1, 0, 0) x (0, 0, -1)
ref_plane "to_ball3_34_ZX" through (2.55, 12.5, 143) normal (0, 0, -1) x (0, 1, 0)
ref_plane "to_ball3_35_XY" through (2.55, 12.5, 139.2) normal (0, 1, 0) x (1, 0, 0)
ref_plane "to_ball3_35_YZ" through (2.55, 12.5, 139.2) normal (1, 0, 0) x (0, 0, -1)
ref_plane "to_ball3_35_ZX" through (2.55, 12.5, 139.2) normal (0, 0, -1) x (0, 1, 0)
ref_plane "to_ball3_36_XY" through (2.55, 12.5, 135.4) normal (0, 1, 0) x (1, 0, 0)
ref_plane "to_ball3_36_YZ" through (2.55, 12.5, 135.4) normal (1, 0, 0) x (0, 0, -1)
ref_plane "to_ball3_36_ZX" through (2.55, 12.5, 135.4) normal (0, 0, -1) x (0, 1, 0)
ref_plane "to_ball3_37_XY" through (2.55, 12.5, 131.6) normal (0, 1, 0) x (1, 0, 0)
ref_plane "to_ball3_37_YZ" through (2.55, 12.5, 131.6) normal (1, 0, 0) x (0, 0, -1)
ref_plane "to_ball3_37_ZX" through (2.55, 12.5, 131.6) normal (0, 0, -1) x (0, 1, 0)
ref_plane "to_ball3_4_XY" through (2.55, 12.5, 257) normal (0, 1, 0) x (1, 0, 0)
ref_plane "to_ball3_4_YZ" through (2.55, 12.5, 257) normal (1, 0, 0) x (0, 0, -1)
ref_plane "to_ball3_4_ZX" through (2.55, 12.5, 257) normal (0, 0, -1) x (0, 1, 0)
ref_plane "to_ball3_5_XY" through (2.55, 12.5, 253.2) normal (0, 1, 0) x (1, 0, 0)
ref_plane "to_ball3_5_YZ" through (2.55, 12.5, 253.2) normal (1, 0, 0) x (0, 0, -1)
ref_plane "to_ball3_5_ZX" through (2.55, 12.5, 253.2) normal (0, 0, -1) x (0, 1, 0)
ref_plane "to_ball3_6_XY" through (2.55, 12.5, 249.4) normal (0, 1, 0) x (1, 0, 0)
ref_plane "to_ball3_6_YZ" through (2.55, 12.5, 249.4) normal (1, 0, 0) x (0, 0, -1)
ref_plane "to_ball3_6_ZX" through (2.55, 12.5, 249.4) normal (0, 0, -1) x (0, 1, 0)
ref_plane "to_ball3_7_XY" through (2.55, 12.5, 245.6) normal (0, 1, 0) x (1, 0, 0)
ref_plane "to_ball3_7_YZ" through (2.55, 12.5, 245.6) normal (1, 0, 0) x (0, 0, -1)
ref_plane "to_ball3_7_ZX" through (2.55, 12.5, 245.6) normal (0, 0, -1) x (0, 1, 0)
ref_plane "to_ball3_8_XY" through (2.55, 12.5, 241.8) normal (0, 1, 0) x (1, 0, 0)
ref_plane "to_ball3_8_YZ" through (2.55, 12.5, 241.8) normal (1, 0, 0) x (0, 0, -1)
ref_plane "to_ball3_8_ZX" through (2.55, 12.5, 241.8) normal (0, 0, -1) x (0, 1, 0)
ref_plane "to_ball3_9_XY" through (2.55, 12.5, 238) normal (0, 1, 0) x (1, 0, 0)
ref_plane "to_ball3_9_YZ" through (2.55, 12.5, 238) normal (1, 0, 0) x (0, 0, -1)
ref_plane "to_ball3_9_ZX" through (2.55, 12.5, 238) normal (0, 0, -1) x (0, 1, 0)
ref_plane "to_ball4_1_XY" through (8.85, 12.5, 268.4) normal (0, 1, 0) x (1, 0, 0)
ref_plane "to_ball4_1_YZ" through (8.85, 12.5, 268.4) normal (1, 0, 0) x (0, 0, -1)
ref_plane "to_ball4_1_ZX" through (8.85, 12.5, 268.4) normal (0, 0, -1) x (0, 1, 0)
ref_plane "to_ball4_10_XY" through (8.85, 12.5, 234.2) normal (0, 1, 0) x (1, 0, 0)
ref_plane "to_ball4_10_YZ" through (8.85, 12.5, 234.2) normal (1, 0, 0) x (0, 0, -1)
ref_plane "to_ball4_10_ZX" through (8.85, 12.5, 234.2) normal (0, 0, -1) x (0, 1, 0)
ref_plane "to_ball4_11_XY" through (8.85, 12.5, 230.4) normal (0, 1, 0) x (1, 0, 0)
ref_plane "to_ball4_11_YZ" through (8.85, 12.5, 230.4) normal (1, 0, 0) x (0, 0, -1)
ref_plane "to_ball4_11_ZX" through (8.85, 12.5, 230.4) normal (0, 0, -1) x (0, 1, 0)
ref_plane "to_ball4_12_XY" through (8.85, 12.5, 226.6) normal (0, 1, 0) x (1, 0, 0)
ref_plane "to_ball4_12_YZ" through (8.85, 12.5, 226.6) normal (1, 0, 0) x (0, 0, -1)
ref_plane "to_ball4_12_ZX" through (8.85, 12.5, 226.6) normal (0, 0, -1) x (0, 1, 0)
ref_plane "to_ball4_13_XY" through (8.85, 12.5, 222.8) normal (0, 1, 0) x (1, 0, 0)
ref_plane "to_ball4_13_YZ" through (8.85, 12.5, 222.8) normal (1, 0, 0) x (0, 0, -1)
ref_plane "to_ball4_13_ZX" through (8.85, 12.5, 222.8) normal (0, 0, -1) x (0, 1, 0)
ref_plane "to_ball4_14_XY" through (8.85, 12.5, 219) normal (0, 1, 0) x (1, 0, 0)
ref_plane "to_ball4_14_YZ" through (8.85, 12.5, 219) normal (1, 0, 0) x (0, 0, -1)
ref_plane "to_ball4_14_ZX" through (8.85, 12.5, 219) normal (0, 0, -1) x (0, 1, 0)
ref_plane "to_ball4_15_XY" through (8.85, 12.5, 215.2) normal (0, 1, 0) x (1, 0, 0)
ref_plane "to_ball4_15_YZ" through (8.85, 12.5, 215.2) normal (1, 0, 0) x (0, 0, -1)
ref_plane "to_ball4_15_ZX" through (8.85, 12.5, 215.2) normal (0, 0, -1) x (0, 1, 0)
ref_plane "to_ball4_16_XY" through (8.85, 12.5, 211.4) normal (0, 1, 0) x (1, 0, 0)
ref_plane "to_ball4_16_YZ" through (8.85, 12.5, 211.4) normal (1, 0, 0) x (0, 0, -1)
ref_plane "to_ball4_16_ZX" through (8.85, 12.5, 211.4) normal (0, 0, -1) x (0, 1, 0)
ref_plane "to_ball4_17_XY" through (8.85, 12.5, 207.6) normal (0, 1, 0) x (1, 0, 0)
ref_plane "to_ball4_17_YZ" through (8.85, 12.5, 207.6) normal (1, 0, 0) x (0, 0, -1)
ref_plane "to_ball4_17_ZX" through (8.85, 12.5, 207.6) normal (0, 0, -1) x (0, 1, 0)
ref_plane "to_ball4_18_XY" through (8.85, 12.5, 203.8) normal (0, 1, 0) x (1, 0, 0)
ref_plane "to_ball4_18_YZ" through (8.85, 12.5, 203.8) normal (1, 0, 0) x (0, 0, -1)
ref_plane "to_ball4_18_ZX" through (8.85, 12.5, 203.8) normal (0, 0, -1) x (0, 1, 0)
ref_plane "to_ball4_19_XY" through (8.85, 12.5, 200) normal (0, 1, 0) x (1, 0, 0)
ref_plane "to_ball4_19_YZ" through (8.85, 12.5, 200) normal (1, 0, 0) x (0, 0, -1)
ref_plane "to_ball4_19_ZX" through (8.85, 12.5, 200) normal (0, 0, -1) x (0, 1, 0)
ref_plane "to_ball4_2_XY" through (8.85, 12.5, 264.6) normal (0, 1, 0) x (1, 0, 0)
ref_plane "to_ball4_2_YZ" through (8.85, 12.5, 264.6) normal (1, 0, 0) x (0, 0, -1)
ref_plane "to_ball4_2_ZX" through (8.85, 12.5, 264.6) normal (0, 0, -1) x (0, 1, 0)
ref_plane "to_ball4_20_XY" through (8.85, 12.5, 196.2) normal (0, 1, 0) x (1, 0, 0)
ref_plane "to_ball4_20_YZ" through (8.85, 12.5, 196.2) normal (1, 0, 0) x (0, 0, -1)
ref_plane "to_ball4_20_ZX" through (8.85, 12.5, 196.2) normal (0, 0, -1) x (0, 1, 0)
ref_plane "to_ball4_21_XY" through (8.85, 12.5, 192.4) normal (0, 1, 0) x (1, 0, 0)
ref_plane "to_ball4_21_YZ" through (8.85, 12.5, 192.4) normal (1, 0, 0) x (0, 0, -1)
ref_plane "to_ball4_21_ZX" through (8.85, 12.5, 192.4) normal (0, 0, -1) x (0, 1, 0)
ref_plane "to_ball4_22_XY" through (8.85, 12.5, 188.6) normal (0, 1, 0) x (1, 0, 0)
ref_plane "to_ball4_22_YZ" through (8.85, 12.5, 188.6) normal (1, 0, 0) x (0, 0, -1)
ref_plane "to_ball4_22_ZX" through (8.85, 12.5, 188.6) normal (0, 0, -1) x (0, 1, 0)
ref_plane "to_ball4_23_XY" through (8.85, 12.5, 184.8) normal (0, 1, 0) x (1, 0, 0)
ref_plane "to_ball4_23_YZ" through (8.85, 12.5, 184.8) normal (1, 0, 0) x (0, 0, -1)
ref_plane "to_ball4_23_ZX" through (8.85, 12.5, 184.8) normal (0, 0, -1) x (0, 1, 0)
ref_plane "to_ball4_24_XY" through (8.85, 12.5, 181) normal (0, 1, 0) x (1, 0, 0)
ref_plane "to_ball4_24_YZ" through (8.85, 12.5, 181) normal (1, 0, 0) x (0, 0, -1)
ref_plane "to_ball4_24_ZX" through (8.85, 12.5, 181) normal (0, 0, -1) x (0, 1, 0)
ref_plane "to_ball4_25_XY" through (8.85, 12.5, 177.2) normal (0, 1, 0) x (1, 0, 0)
ref_plane "to_ball4_25_YZ" through (8.85, 12.5, 177.2) normal (1, 0, 0) x (0, 0, -1)
ref_plane "to_ball4_25_ZX" through (8.85, 12.5, 177.2) normal (0, 0, -1) x (0, 1, 0)
ref_plane "to_ball4_26_XY" through (8.85, 12.5, 173.4) normal (0, 1, 0) x (1, 0, 0)
ref_plane "to_ball4_26_YZ" through (8.85, 12.5, 173.4) normal (1, 0, 0) x (0, 0, -1)
ref_plane "to_ball4_26_ZX" through (8.85, 12.5, 173.4) normal (0, 0, -1) x (0, 1, 0)
ref_plane "to_ball4_27_XY" through (8.85, 12.5, 169.6) normal (0, 1, 0) x (1, 0, 0)
ref_plane "to_ball4_27_YZ" through (8.85, 12.5, 169.6) normal (1, 0, 0) x (0, 0, -1)
ref_plane "to_ball4_27_ZX" through (8.85, 12.5, 169.6) normal (0, 0, -1) x (0, 1, 0)
ref_plane "to_ball4_28_XY" through (8.85, 12.5, 165.8) normal (0, 1, 0) x (1, 0, 0)
ref_plane "to_ball4_28_YZ" through (8.85, 12.5, 165.8) normal (1, 0, 0) x (0, 0, -1)
ref_plane "to_ball4_28_ZX" through (8.85, 12.5, 165.8) normal (0, 0, -1) x (0, 1, 0)
ref_plane "to_ball4_29_XY" through (8.85, 12.5, 162) normal (0, 1, 0) x (1, 0, 0)
ref_plane "to_ball4_29_YZ" through (8.85, 12.5, 162) normal (1, 0, 0) x (0, 0, -1)
ref_plane "to_ball4_29_ZX" through (8.85, 12.5, 162) normal (0, 0, -1) x (0, 1, 0)
ref_plane "to_ball4_3_XY" through (8.85, 12.5, 260.8) normal (0, 1, 0) x (1, 0, 0)
ref_plane "to_ball4_3_YZ" through (8.85, 12.5, 260.8) normal (1, 0, 0) x (0, 0, -1)
ref_plane "to_ball4_3_ZX" through (8.85, 12.5, 260.8) normal (0, 0, -1) x (0, 1, 0)
ref_plane "to_ball4_30_XY" through (8.85, 12.5, 158.2) normal (0, 1, 0) x (1, 0, 0)
ref_plane "to_ball4_30_YZ" through (8.85, 12.5, 158.2) normal (1, 0, 0) x (0, 0, -1)
ref_plane "to_ball4_30_ZX" through (8.85, 12.5, 158.2) normal (0, 0, -1) x (0, 1, 0)
ref_plane "to_ball4_31_XY" through (8.85, 12.5, 154.4) normal (0, 1, 0) x (1, 0, 0)
ref_plane "to_ball4_31_YZ" through (8.85, 12.5, 154.4) normal (1, 0, 0) x (0, 0, -1)
ref_plane "to_ball4_31_ZX" through (8.85, 12.5, 154.4) normal (0, 0, -1) x (0, 1, 0)
ref_plane "to_ball4_32_XY" through (8.85, 12.5, 150.6) normal (0, 1, 0) x (1, 0, 0)
ref_plane "to_ball4_32_YZ" through (8.85, 12.5, 150.6) normal (1, 0, 0) x (0, 0, -1)
ref_plane "to_ball4_32_ZX" through (8.85, 12.5, 150.6) normal (0, 0, -1) x (0, 1, 0)
ref_plane "to_ball4_33_XY" through (8.85, 12.5, 146.8) normal (0, 1, 0) x (1, 0, 0)
ref_plane "to_ball4_33_YZ" through (8.85, 12.5, 146.8) normal (1, 0, 0) x (0, 0, -1)
ref_plane "to_ball4_33_ZX" through (8.85, 12.5, 146.8) normal (0, 0, -1) x (0, 1, 0)
ref_plane "to_ball4_34_XY" through (8.85, 12.5, 143) normal (0, 1, 0) x (1, 0, 0)
ref_plane "to_ball4_34_YZ" through (8.85, 12.5, 143) normal (1, 0, 0) x (0, 0, -1)
ref_plane "to_ball4_34_ZX" through (8.85, 12.5, 143) normal (0, 0, -1) x (0, 1, 0)
ref_plane "to_ball4_35_XY" through (8.85, 12.5, 139.2) normal (0, 1, 0) x (1, 0, 0)
ref_plane "to_ball4_35_YZ" through (8.85, 12.5, 139.2) normal (1, 0, 0) x (0, 0, -1)
ref_plane "to_ball4_35_ZX" through (8.85, 12.5, 139.2) normal (0, 0, -1) x (0, 1, 0)
ref_plane "to_ball4_36_XY" through (8.85, 12.5, 135.4) normal (0, 1, 0) x (1, 0, 0)
ref_plane "to_ball4_36_YZ" through (8.85, 12.5, 135.4) normal (1, 0, 0) x (0, 0, -1)
ref_plane "to_ball4_36_ZX" through (8.85, 12.5, 135.4) normal (0, 0, -1) x (0, 1, 0)
ref_plane "to_ball4_37_XY" through (8.85, 12.5, 131.6) normal (0, 1, 0) x (1, 0, 0)
ref_plane "to_ball4_37_YZ" through (8.85, 12.5, 131.6) normal (1, 0, 0) x (0, 0, -1)
ref_plane "to_ball4_37_ZX" through (8.85, 12.5, 131.6) normal (0, 0, -1) x (0, 1, 0)
ref_plane "to_ball4_4_XY" through (8.85, 12.5, 257) normal (0, 1, 0) x (1, 0, 0)
ref_plane "to_ball4_4_YZ" through (8.85, 12.5, 257) normal (1, 0, 0) x (0, 0, -1)
ref_plane "to_ball4_4_ZX" through (8.85, 12.5, 257) normal (0, 0, -1) x (0, 1, 0)
ref_plane "to_ball4_5_XY" through (8.85, 12.5, 253.2) normal (0, 1, 0) x (1, 0, 0)
ref_plane "to_ball4_5_YZ" through (8.85, 12.5, 253.2) normal (1, 0, 0) x (0, 0, -1)
ref_plane "to_ball4_5_ZX" through (8.85, 12.5, 253.2) normal (0, 0, -1) x (0, 1, 0)
ref_plane "to_ball4_6_XY" through (8.85, 12.5, 249.4) normal (0, 1, 0) x (1, 0, 0)
ref_plane "to_ball4_6_YZ" through (8.85, 12.5, 249.4) normal (1, 0, 0) x (0, 0, -1)
ref_plane "to_ball4_6_ZX" through (8.85, 12.5, 249.4) normal (0, 0, -1) x (0, 1, 0)
ref_plane "to_ball4_7_XY" through (8.85, 12.5, 245.6) normal (0, 1, 0) x (1, 0, 0)
ref_plane "to_ball4_7_YZ" through (8.85, 12.5, 245.6) normal (1, 0, 0) x (0, 0, -1)
ref_plane "to_ball4_7_ZX" through (8.85, 12.5, 245.6) normal (0, 0, -1) x (0, 1, 0)
ref_plane "to_ball4_8_XY" through (8.85, 12.5, 241.8) normal (0, 1, 0) x (1, 0, 0)
ref_plane "to_ball4_8_YZ" through (8.85, 12.5, 241.8) normal (1, 0, 0) x (0, 0, -1)
ref_plane "to_ball4_8_ZX" through (8.85, 12.5, 241.8) normal (0, 0, -1) x (0, 1, 0)
ref_plane "to_ball4_9_XY" through (8.85, 12.5, 238) normal (0, 1, 0) x (1, 0, 0)
ref_plane "to_ball4_9_YZ" through (8.85, 12.5, 238) normal (1, 0, 0) x (0, 0, -1)
ref_plane "to_ball4_9_ZX" through (8.85, 12.5, 238) normal (0, 0, -1) x (0, 1, 0)
ref_plane "to_body_XY" through (5.7, 6.05, 200) normal (0, 0, 1) x (1, 0, 0)
ref_plane "to_body_YZ" through (5.7, 6.05, 200) normal (1, 0, 0) x (0, 1, 0)
ref_plane "to_body_ZX" through (5.7, 6.05, 200) normal (0, 1, 0) x (0, 0, 1)
ref_plane "to_body2_XY" through (5.7, 6.05, 200) normal (0, 0, 1) x (1, 0, 0)
ref_plane "to_body2_YZ" through (5.7, 6.05, 200) normal (1, 0, 0) x (0, 1, 0)
ref_plane "to_body2_ZX" through (5.7, 6.05, 200) normal (0, 1, 0) x (0, 0, 1)
body "Solid1"
